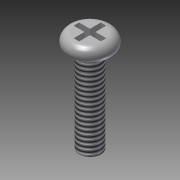
# Autodesk Inventor part: screw_M2_8
Saved by Autodesk Inventor 2013 (Build 170138000, 138)
## iProperties
Shininess: 50.0
Created: 2011-05-14
Part Number: screw_M2_8
Document SubType Name: Modeling
Designer: Noa Izumi
Material: Default
Density: 1 g/cm^3
Density: 0.0
Volumn: 0.0
Area: 0.0
PropertySet Name: Model Information
Control State: 0
Master: False
Checked Out: False
Author: Noa Izumi
Autodesk Inventor part; units mm, degrees
ref_plane "YZ Plane" through (0, 0, 0) normal (1, 0, 0) x (0, 1, 0)
ref_plane "XZ Plane" through (0, 0, 0) normal (0, 1, 0) x (-1, 0, 0)
ref_plane "XY Plane" through (0, 0, 0) normal (0, 0, 1) x (1, 0, 0)
sketch "Sketch1" plane through (0, 0, 0) normal (0, 0, 1) x (1, 0, 0)
  circle A0 centre (0, 0) radius 2
  dimension "d0" = 4
  constraints: 1 centre point
  measures "d0" diameter of A0
extrude "Extrusion1" add sketch "Sketch1" along normal blind 1.25
fillet "Fillet1" radius 0.5 1 edges at (-2, 0, 0)
fillet "Fillet2" radius 0.75 1 edges at (-2, 0, 1.25)
sketch "Sketch2" plane through (0, 0, 1.25) normal (0, 0, 1) x (1, 0, 0)
  line L0 (-1.25, -0.2499) -> (-1.25, 0.2501)
  line L1 (-1.25, 0.2501) -> (-0.25, 0.2501)
  line L2 (-0.25, 0.2501) -> (-0.25, 1.2501)
  line L3 (-0.25, 1.2501) -> (0.25, 1.2501)
  line L4 (0.25, 1.2501) -> (0.25, 0.2501)
  line L5 (0.25, 0.2501) -> (1.25, 0.2501)
  line L6 (1.25, 0.2501) -> (1.25, -0.2499)
  line L7 (1.25, -0.2499) -> (0.25, -0.2499)
  line L8 (0.25, -0.2499) -> (0.25, -1.2499)
  line L9 (0.25, -1.2499) -> (-0.25, -1.2499)
  line L10 (-0.25, -1.2499) -> (-0.25, -0.2499)
  line L11 (-0.25, -0.2499) -> (-1.25, -0.2499)
  dimension "d24" = 0.5
  dimension "d27" = 0.5
  dimension "d28" = 0.5
  dimension "d29" = 0.5
  dimension "d30" = 1
  dimension "d31" = 1
  dimension "d32" = 1
  dimension "d33" = 1
  dimension "d34" = 1
  dimension "d35" = 1
  constraints: 24 end point, 10 parallel, 4 perpendicular
  measures "d24" distance of L0.start L0.end
  measures "d27" distance of L5.end L6.end
  measures "d28" distance of L2.end L3.end
  measures "d29" distance of L8.end L9.end
  measures "d30" distance of L10.end L0.start
  measures "d31" distance of L6.end L7.end
  measures "d32" distance of L0.end L1.end
  measures "d33" distance of L1.end L2.end
  measures "d34" distance of L9.end L10.end
  measures "d35" distance of L3.end L4.end
extrude "Extrusion2" cut sketch "Sketch2" against normal blind 1
sketch "Sketch3" plane through (0, 0, 0) normal (0, 0, -1) x (-1, 0, 0)
  circle A0 centre (0, 0) radius 1.5 projected
  circle A1 centre (0, 0) radius 1
  dimension "d19" = 2
  constraints: 1 centre point, 1 coincident
  measures "d19" diameter of A1
extrude "Extrusion3" add sketch "Sketch3" along normal blind 8 contours A1
chamfer "Chamfer3" distance 0.5 angle 45 4 edges at (-1.25, 0.0001, 0.25) (0, 1.2501, 0.25) (0, -1.2499, 0.25) (1.25, 0.0001, 0.25)
thread "Thread2" size "M2x0.4" class "6g" standard "ANSI Metric M Profile" full length
